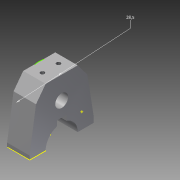
# Autodesk Inventor part: 2DOF-150-18-LEVS-01
Saved by Autodesk Inventor 2013 (Build 170138000, 138)
## iProperties
Company: Simumak
Created: 2013-09-16
Part Number: 2DOF-150-18-LEVS-01
Material: Stainless Steel
Document SubType Name: Modeling
Designer: Yolanda Garrido
Density: 8.08 g/cm^3
Mass: 104.72 g
Surface Area: 50.1751 cm^2
Volume: 12.9604 cm^3
Project: 2DOF-150-ASI
Description: Parte superior de la leva
Stock Number: 1702
Author: Yolanda Garrido
Title: Parte superior de la leva
Comments: Pavonado
Autodesk Inventor part; units mm, degrees
ref_plane "YZ Plane" through (0, 0, 0) normal (1, 0, 0) x (0, 1, 0)
sketch "Sketch1" plane through (0, 0, 0) normal (1, 0, 0) x (0, 1, 0)
  circle A0 centre (0, 0) radius 4
  line L0 (0, 0) -> (0, -22) construction
  line L1 (-10, -22) -> (-20, -22)
  line L2 (-20, -22) -> (-20, -19.8078)
  line L3 (10, -22) -> (20, -22)
  line L4 (20, -22) -> (20, -19.6315)
  line L5 (0, -9.2) -> (3, -9.2)
  line L6 (3, -9.2) -> (3, -12.4606)
  line L7 (0, -9.2) -> (-3, -9.2)
  line L8 (-3, -9.2) -> (-3, -12.4606)
  arc A1 (10, -22) -> (3, -12.4606) centre (0, -22) ccw
  arc A2 (-3, -12.4606) -> (-10, -22) centre (0, -22) ccw
  arc A3 (-19.9864, -19.6315) -> (-20, -19.8078) centre (-18.8527, -19.8078) ccw
  arc A4 (20, -19.6315) -> (19.8774, -18.0974) centre (10.3433, -19.6315) ccw
  line L9 (-19.9864, -19.6315) -> (-16, 6)
  line L10 (16, 6) -> (19.8774, -18.0974)
  line L11 (0, 14) -> (-10, 14)
  line L12 (-10, 14) -> (-16, 6)
  line L13 (0, 14) -> (10, 14)
  line L14 (10, 14) -> (16, 6)
  point P0 (-20, -12)
  point P1 (20, -12)
  dimension "d0" = 8
  dimension "d2" = 22
  dimension "d4" = 20
  dimension "d5" = 10
  dimension "d13" = 12.8
  dimension "d26" = 10
  dimension "d73" = 10
  dimension "d74" = 8
  dimension "d76" = 10
  dimension "d107" = 6
  dimension "d119" = 6
  dimension "d122" = 14
  constraints: 30 end point, 8 point on circle, 7 symmetric about line, 5 centre point, 4 point on line, 4 tangent, 3 coincident, 3 perpendicular, 1 parallel, 1 vertical
  measures "d0" diameter of A0
  measures "d2" distance of L0.start L0.end
  measures "d4" distance of A1.centre L1.end
  measures "d5" distance of L1.end point (-20, -12)
  measures "d13" distance between parallel lines of L3 L5
  measures "d26" radius of A1
  measures "d73" distance of L11.start L11.end
  measures "d74" vertical distance of L9.end L11.end
  measures "d76" distance of L14.start L11.start
  measures "d107" distance between parallel lines of L6 L8
  measures "d119" horizontal distance of L11.end L9.end
  measures "d122" distance from line of point (0, 0) L13
extrude "Extrusion1" add sketch "Sketch1" along normal mid plane 14
sketch "Sketch2" plane through (7, -10, -22) normal (0, 0, -1) x (-1, 0, 0)
  line L0 (14, 0) -> (14, -10) projected
  line L1 (7, 10) -> (-4.9056, 10) construction
  line L2 (14, 20) -> (0, 20)
  line L3 (0, 30) -> (0, 20)
  line L4 (0, 30) -> (14, 30)
  line L5 (14, 20) -> (14, 30)
  line L6 (0, -10) -> (0, 0) projected
  line L7 (14, 0) -> (0, 0) projected
  line L8 (0, -10) -> (14, -10) projected
  point P0 (5, 26.5)
  point P1 (5, -6.5)
  dimension "d46" = 5
  dimension "d48" = 3.5
  dimension "d50" = 5
  dimension "d51" = 3.5
  constraints: 10 end point, 4 symmetric about line, 1 perpendicular
  measures "d46" distance from line of L3 point (5, 26.5)
  measures "d48" distance from line of L4 point (5, 26.5)
  measures "d50" distance from line of point (5, -6.5) L6
  measures "d51" vertical distance of L6.start point (5, -6.5)
ref_plane "Work Plane1" through (16, 0, 0) normal (1, 0, 0) x (0, 0, -1)
sketch "Sketch7" plane through (-7, 0, 0) normal (-1, 0, 0) x (0, 0, 1)
  circle A0 centre (0, 0) radius 4 projected
  circle A1 centre (0, 0) radius 14.25
  dimension "d52" = 28.5
  constraints: 1 centre point
  measures "d52" diameter of A1
sketch "Sketch10" plane through (-7, -10, 14) normal (0, 0, 1) x (1, 0, 0)
  line L0 (0, 0) -> (14, 0) projected
  line L1 (14, 20) -> (14, 0) projected
  line L2 (0, 20) -> (14, 20) projected
  line L3 (0, 0) -> (0, 20) projected
  point P0 (7, 10)
sketch "Sketch15" plane through (7, -10, -22) normal (0, 0, -1) x (-1, 0, 0)
  line L0 (14, 0) -> (0, 0) projected
  line L1 (0, -10) -> (0, 0) projected
  line L2 (0, -10) -> (14, -10) projected
  line L3 (14, 0) -> (14, -10) projected
  point P0 (7, 10)
sketch "Sketch16" plane through (7, -10, -22) normal (0, 0, -1) x (-1, 0, 0)
  line L0 (0, -10) -> (14, -10) projected
  line L1 (14, 0) -> (14, -10) projected
  line L2 (7, -10) -> (7, 30.0311)
  line L3 (4.3309, -5) -> (12.7149, -5)
  line L4 (3.2036, 25) -> (11.1649, 25)
  line L5 (14, 30) -> (0, 30) projected
  line L6 (0, 20) -> (0, 30) projected
  line L7 (14, 20) -> (0, 20) projected
  line L8 (14, 30) -> (14, 20) projected
  point P0 (7, 10)
  point P1 (7, 25)
  point P2 (7, -5)
  dimension "d110" = 5
  dimension "d111" = 5
  constraints: 6 end point, 4 point on line, 2 parallel, 1 midpoint, 1 perpendicular
  measures "d110" distance between parallel lines of L4 L5
  measures "d111" distance between parallel lines of L0 L3
hole "Hole13" at (0, -15, -22) at (0, 15, -22) direction (0, 0, 1) diameter 4.134 depth 13.5 tip angle 118 thread size "M5x0.8" class "6H" standard "ANSI Metric M Profile"
ref_plane "Work Plane2" through (19.5, 0, 0) normal (1, 0, 0) x (0, 0, -1)
sketch "Sketch17" plane through (19.5, 0, 0) normal (1, 0, 0) x (0, 0, -1)
  point P0 (0, 0)
  point P1 (0, 0)
  constraints: 1 coincident
sketch "Sketch18" plane through (-7, -10, 14) normal (0, 0, 1) x (1, 0, 0)
  circle A0 centre (7, 15) radius 1.5
  line L0 (0, 0) -> (14, 0) projected
  line L1 (14, 20) -> (14, 0) projected
  line L2 (0, 20) -> (14, 20) projected
  line L3 (0, 0) -> (0, 20) projected
  circle A1 centre (7, 5) radius 1.5
  point P0 (7, 10)
  dimension "d132" = 7
  constraints: 2 centre point, 1 vertical alignment
  measures "d132" distance from line of L3 A0.centre
hole "Hole14" at (0, 5, 14) at (0, -5, 14) direction (0, 0, -1) diameter 2.459 depth 6.5 tip angle 118 thread size "M3x0.5" class "6H" standard "ANSI Metric M Profile"
equation "\"d46\" = d50"
equation "\"d51\" = d48"
body "Solid1"
